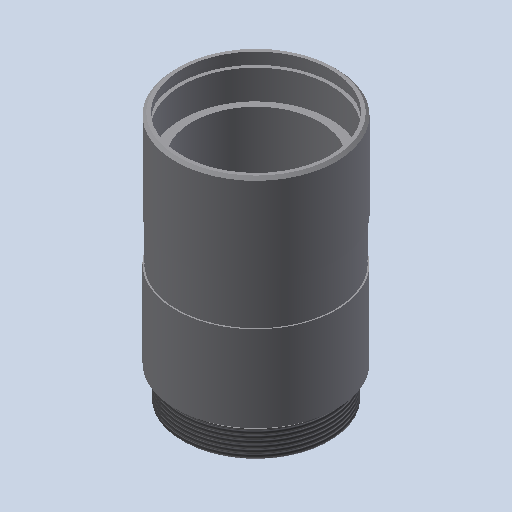
# Autodesk Inventor part: Lampengehäuse
Saved by Autodesk Inventor 2022 (Build 260153000, 153)
## iProperties
Created: 2014-03-26
Part Number: Lampengehäuse
Material: Generisch
Document SubType Name: Modeling
Designer: G. Schardt
Density: 1 g/cm^3
Appearance: Vorgabe
Mass: 75.4577 g
Surface Area: 329.038 cm^2
Volume: 75.4577 cm^3
Project: 10W LED Lampenkopf
Author: demo.user
Autodesk Inventor part; units mm, degrees
sketch "Skizze1" plane through (0, 0, 0) normal (0, 0, 1) x (1, 0, 0)
  circle A0 centre (0, 0) radius 30
  dimension "d0" = 60
  constraints: 1 centre point, 1 coincident
  measures "d0" diameter of A0
extrude "Extrusion1" add sketch "Skizze1" along normal mid plane 93
ref_plane "Arbeitsebene1" through (0, 0, 13.5) normal (0, 0, 1) x (1, 0, 0)
ref_plane "Arbeitsebene2" through (0, 0, -2.5) normal (0, 0, 1) x (1, 0, 0)
ref_plane "Arbeitsebene11" through (0, 0, 45) normal (0, 0, 1) x (1, 0, 0)
sketch "Skizze12" plane through (0, 0, 13.5) normal (0, 0, 1) x (1, 0, 0)
  circle A0 centre (0, 0) radius 29.5
  circle A1 centre (0, 0) radius 30 projected
  dimension "d91" = 0.5
  constraints: 1 centre point
  measures "d91" radial gap between concentric circles of A0 A1
extrude "Extrusion9" cut sketch "Skizze12" against normal up to surface (16 mm away)
sketch "Skizze3" plane through (0, 0, 46.5) normal (0, 0, 1) x (1, 0, 0)
  point P0 (0, 0)
  point P1 (0, 0)
  constraints: 1 coincident
hole "Bohrung1" at (0, 0, 46.5) direction (0, 0, -1) diameter 55.5 depth 15
ref_plane "Arbeitsebene13" through (0, 0, 33) normal (0, 0, 1) x (1, 0, 0)
sketch "Skizze4" plane through (0, 0, 31.5) normal (0, 0, 1) x (1, 0, 0)
  point P0 (0, 0)
  point P1 (0, 0)
  constraints: 1 coincident
hole "Bohrung2" at (0, 0, 31.5) direction (0, 0, -1) diameter 47.5 end through all
sketch "Skizze5" plane through (0, 0, -46.5) normal (0, 0, -1) x (-1, 0, 0)
  point P0 (0, 0)
  point P1 (0, 0)
  constraints: 1 coincident
hole "Bohrung3" at (0, 0, -46.5) direction (0, 0, 1) diameter 49 depth 43
sketch "Skizze6" plane through (0, 0, -46.5) normal (0, 0, -1) x (-1, 0, 0)
  circle A0 centre (0, 0) radius 27.5
  circle A1 centre (0, 0) radius 30 projected
  dimension "d35" = 55
  constraints: 1 centre point, 1 coincident
  measures "d35" diameter of A0
extrude "Extrusion3" cut sketch "Skizze6" against normal blind 12
ref_plane "Arbeitsebene4" through (0, 0, -36.5) normal (0, 0, -1) x (-1, 0, 0)
sketch "Skizze7" plane through (0, 0, -46.5) normal (0, 0, -1) x (-1, 0, 0)
  circle A0 centre (0, 0) radius 26.6
  circle A1 centre (0, 0) radius 27.5 projected
  dimension "d39" = 53.2
  constraints: 1 centre point, 1 coincident
  measures "d39" diameter of A0
ref_plane "Arbeitsebene5" through (0, 0, -34.5) normal (0, 0, -1) x (-1, 0, 0)
extrude "Extrusion4" cut sketch "Skizze7" along normal up to surface (2 mm away) from surface at -12
thread "Gewinde1" size "M55x1.5" class "6g" standard "ISO Metric profile" full length
chamfer "Fase3" distance 0.5 angle 45 1 edges at (27.5, 0, -46.5)
ref_plane "Arbeitsebene10" through (0, 0, -8.4) normal (0, 0, -1) x (-1, 0, 0)
ref_plane "Arbeitsebene9" through (0, 0, -5.5) normal (0, 0, -1) x (-1, 0, 0)
sketch "Skizze9" plane through (0, 0, -8.4) normal (0, 0, -1) x (-1, 0, 0)
  circle A0 centre (0, 0) radius 25.6
  dimension "d67" = 51.2
  constraints: 1 centre point, 1 coincident
  measures "d67" diameter of A0
extrude "Extrusion6" cut sketch "Skizze9" against normal up to surface (2.9 mm away) from surface at 0
chamfer "Fase8" distance 1 angle 45 1 edges at (0, -24.5, -46.5)
ref_plane "Arbeitsebene12" through (0, 0, 33) normal (0, 0, 1) x (1, 0, 0)
sketch "Skizze10" plane through (0, 0, 31.5) normal (0, 0, 1) x (1, 0, 0)
  circle A0 centre (0, 0) radius 23.75 projected
  circle A1 centre (0, 0) radius 25.25
  circle A2 centre (0, 0) radius 27.75
  circle A3 centre (0, 0) radius 27.75 projected
  dimension "d76" = 1.5
  dimension "d77" = 2.5
  constraints: 2 centre point
  measures "d76" radial gap between concentric circles of A0 A1
  measures "d77" radial gap between concentric circles of A1 A2
extrude "Extrusion7" cut sketch "Skizze10" against normal blind 1.1 contours A2
ref_plane "Arbeitsebene14" through (0, 0, 41.3) normal (0, 0, 1) x (1, 0, 0)
sketch "Skizze11" plane through (0, 0, 41.3) normal (0, 0, 1) x (1, 0, 0)
  circle A0 centre (0, 0) radius 27.75 projected
  circle A1 centre (0, 0) radius 29
  dimension "d82" = 1.25
  constraints: 1 centre point
  measures "d82" radial gap between concentric circles of A0 A1
extrude "Extrusion8" cut sketch "Skizze11" along normal blind 2.4
chamfer "Fase10" distance 1 angle 45 1 edges at (-30, 0, 46.5)
